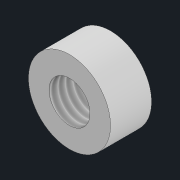
# Autodesk Inventor part: Fijador
Saved by Autodesk Inventor 2021 (Build 250183000, 183)
## iProperties
Created: 2021-05-06
Part Number: Fijador
Material: Generic
Document SubType Name: Modeling
Designer: GABRIEL LOL
Density: 1 g/cm^3
Appearance: Default
Author: GABRIEL LOL
Autodesk Inventor part; units mm, degrees
ref_plane "YZ Plane" through (0, 0, 0) normal (1, 0, 0) x (0, 1, 0)
ref_plane "XZ Plane" through (0, 0, 0) normal (0, 1, 0) x (-1, 0, 0)
ref_plane "XY Plane" through (0, 0, 0) normal (0, 0, 1) x (1, 0, 0)
sketch "Sketch1" plane through (0, 0, 0) normal (0, 0, 1) x (1, 0, 0)
  circle A0 centre (0, 0) radius 1.25
  line L0 (0, 0) -> (0, 2.5) construction
  line L1 (0, 2.5) -> (0, -2.5) construction
  line L2 (0, -2.5) -> (2.5, -2.5) construction
  line L3 (0, 2.5) -> (-2.5, 2.5) construction
  line L4 (2.5, -2.5) -> (-2.5, -2.5)
  line L5 (-2.5, -2.5) -> (-2.5, 2.5)
  line L6 (-2.5, 2.5) -> (2.5, 2.5)
  line L7 (2.5, 2.5) -> (2.5, -2.5)
  dimension "d0" = 2.5
  dimension "d1" = 2.5
  dimension "d2" = 5
  dimension "d3" = 2.5
  dimension "d4" = 2.5
  constraints: 16 end point, 2 horizontal, 2 parallel, 2 perpendicular, 2 vertical, 1 centre point, 1 coincident
  measures "d0" diameter of A0
  measures "d1" distance of L0.start L0.end
  measures "d2" distance of L0.end L1.end
  measures "d3" distance of L1.end L2.end
  measures "d4" distance of L0.end L3.end
extrude "Extrusion1" add sketch "Sketch1" along normal blind 2.5
thread "Thread1" size "M2.5x0.45" class "6H" standard "ANSI Metric M Profile" full length
sketch "Sketch2" plane through (0, 0, 2.5) normal (0, 0, 1) x (1, 0, 0)
  circle A0 centre (0, 0) radius 1.25 projected
  circle A1 centre (0, 0) radius 2.5
  circle A2 centre (0, 0) radius 4.0791
  constraints: 2 centre point, 2 coincident, 1 other
extrude "Extrusion2" cut sketch "Sketch2" against normal blind 10 contours A2
body "Solid1"
